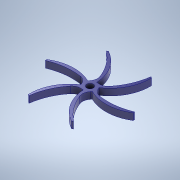
# Autodesk Inventor part: Propelas
Saved by Autodesk Inventor 2020 (Build 240168000, 168)
## iProperties
Created: 2020-10-29
Part Number: Propelas
Material: PC/ABS Plastic
Document SubType Name: Modeling
Designer: aaron
Density: 0.357273 g/cm^3
Appearance: Flaked Satin - Dark Blue
Author: aaron
Autodesk Inventor part; units mm, degrees
ref_plane "YZ Plane" through (0, 0, 0) normal (1, 0, 0) x (0, 1, 0)
ref_plane "XZ Plane" through (0, 0, 0) normal (0, 1, 0) x (-1, 0, 0)
ref_plane "XY Plane" through (0, 0, 0) normal (0, 0, 1) x (1, 0, 0)
sketch "Sketch1" plane through (0, 0, 0) normal (0, 1, 0) x (-1, 0, 0)
  circle A0 centre (0, 0) radius 10 construction
  circle A1 centre (0, 0) radius 1.5
  line L0 (0, 0) -> (4.6947, -8.8295) construction
  line L1 (0, 0) -> (0, -10) construction
  arc A2 (-0.0254, -1.4998) -> (4.6947, -8.8295) centre (8.9547, -0.9015) ccw
  line L2 (0, 0) -> (5, -8.6603) construction
  arc A3 (0.2768, -1.4742) -> (5, -8.6603) centre (12.8599, 1.6512) ccw
  line L3 (4.6947, -8.8295) -> (5, -8.6603)
  arc A4 (-1.3115, -0.7279) -> (-5.2992, -8.4805) centre (3.6966, -8.2058) ccw
  arc A5 (-1.1383, -0.9768) -> (-5, -8.6603) centre (7.8599, -10.3114) ccw
  line L4 (-5.2992, -8.4805) -> (-5, -8.6603)
  arc A6 (-1.2862, 0.7719) -> (-9.9939, 0.349) centre (-5.2581, -7.3043) ccw
  arc A7 (-1.4151, 0.4974) -> (-10, 0) centre (-5, -11.9626) ccw
  line L5 (-9.9939, 0.349) -> (-10, 0)
  arc A8 (0.0254, 1.4998) -> (-4.6947, 8.8295) centre (-8.9547, 0.9015) ccw
  arc A9 (-0.2768, 1.4742) -> (-5, 8.6603) centre (-12.8599, -1.6512) ccw
  line L6 (-4.6947, 8.8295) -> (-5, 8.6603)
  arc A10 (1.3115, 0.7279) -> (5.2992, 8.4805) centre (-3.6966, 8.2058) ccw
  arc A11 (1.1383, 0.9768) -> (5, 8.6603) centre (-7.8599, 10.3114) ccw
  line L7 (5.2992, 8.4805) -> (5, 8.6603)
  arc A12 (1.2862, -0.7719) -> (9.9939, -0.349) centre (5.2581, 7.3043) ccw
  arc A13 (1.4151, -0.4974) -> (10, 0) centre (5, 11.9626) ccw
  line L8 (9.9939, -0.349) -> (10, 0)
  circle A14 centre (0, 0) radius 0.75
  point P0 (1.2862, -0.7719)
  point P1 (1.4151, -0.4974)
  point P2 (1.3115, 0.7279)
  point P3 (1.1383, 0.9768)
  point P4 (0.0254, 1.4998)
  point P5 (-0.2768, 1.4742)
  point P6 (-1.2862, 0.7719)
  point P7 (-1.4151, 0.4974)
  point P8 (-1.3115, -0.7279)
  point P9 (-1.1383, -0.9768)
  dimension "d0" = 20
  dimension "d1" = 3
  dimension "d2" = 28
  dimension "d3" = 9
  dimension "d4" = 30
  dimension "d5" = 0.7
  dimension "d6" = 12.9655
  dimension "d7" = 11.9626
  dimension "d10" = 360
  dimension "d12" = 1.5
  constraints: 29 point on circle, 18 end point, 15 centre point, 3 coincident, 1 vertical, 61 other
  measures "d0" diameter of A0
  measures "d1" diameter of A1
  measures "d2" angle of L1 L0
  measures "d3" radius of A2
  measures "d4" angle of L1 L2
  measures "d6" radius of A3
  measures "d7" distance from line of A3.centre L2
  measures "d12" diameter of A14
extrude "Extrusion1" add sketch "Sketch1" along normal blind 1.5
fillet "Fillet1" radius 2 6 edges at (1.1383, 0.75, -0.9768) (-0.2768, 0.75, -1.4742) (-1.4151, 0.75, -0.4974) (-1.1383, 0.75, 0.9768) (0.2768, 0.75, 1.4742) (1.4151, 0.75, 0.4974)
body "Solid1"
